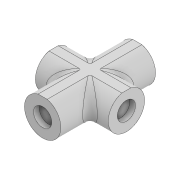
# Autodesk Inventor part: Cross_Minimo
Saved by Autodesk Inventor 2020 (Build 240168000, 168)
## iProperties
Created: 2021-03-31
Part Number: Cross_Minimo
Material: Generic
Document SubType Name: Modeling
Designer: deox
Density: 1 g/cm^3
Appearance: Default
Author: deox
## iProperties of the stored document _3DPrint.ipt
Created: 2021-05-12
Part Number: _3DPrint
Material: Generic
Document SubType Name: Modeling
Designer: deox
Density: 1 g/cm^3
Appearance: Default
Author: deox
Autodesk Inventor part; units mm, degrees
ref_plane "YZ Plane" through (0, 0, 0) normal (1, 0, 0) x (0, 1, 0)
ref_plane "XZ Plane" through (0, 0, 0) normal (0, 1, 0) x (-1, 0, 0)
ref_plane "XY Plane" through (0, 0, 0) normal (0, 0, 1) x (1, 0, 0)
sketch "Sketch1" plane through (0, 0, 0) normal (0, 0, 1) x (1, 0, 0)
  circle A0 centre (0, 0) radius 2.5
  dimension "d0" = 5
  constraints: 1 centre point, 1 coincident
  measures "d0" diameter of A0
extrude "Extrusion1" add sketch "Sketch1" along normal mid plane 13
sketch "Sketch2" plane through (0, 0, 6.5) normal (0, 0, 1) x (1, 0, 0)
  circle A0 centre (0, 0) radius 1.25
  dimension "d3" = 2.5
  constraints: 1 centre point, 1 coincident
  measures "d3" diameter of A0
extrude "Extrusion2" cut sketch "Sketch2" against normal blind 0.8
mirror "Mirror1" about plane through (0, 0, 0) normal (0, 0, 1) of "Extrusion2"
sketch "Sketch3" plane through (0, 0, 0) normal (1, 0, 0) x (0, 1, 0)
  circle A0 centre (0, 0) radius 2.5
  dimension "d6" = 5
  constraints: 1 centre point, 1 coincident
  measures "d6" diameter of A0
extrude "Extrusion3" add sketch "Sketch3" along normal mid plane 10
sketch "Sketch4" plane through (5, 0, 0) normal (1, 0, 0) x (0, 0, -1)
  circle A0 centre (0, 0) radius 1.25
  dimension "d9" = 2.5
  constraints: 1 centre point, 1 coincident
  measures "d9" diameter of A0
extrude "Extrusion4" cut sketch "Sketch4" against normal blind 0.8
mirror "Mirror2" about plane through (0, 0, 0) normal (1, 0, 0) of "Extrusion4"
fillet "Fillet1" radius 1 6 edges at (1.7678, 1.7678, 1.7678) (-2.5, 0, 2.5) (1.7678, -1.7678, 1.7678) (1.7678, -1.7678, -1.7678) (1.7678, 1.7678, -1.7678) (-2.5, 0, -2.5)
sketch "Sketch5" plane through (0, 0, 6.5) normal (0, 0, 1) x (1, 0, 0)
  circle A0 centre (0, 0) radius 2.5 projected
  line L0 (0, 2.5) -> (5.3723, 2.5)
  line L1 (5.3723, 2.5) -> (5.3723, 2.4205)
  line L2 (5.3723, 2.4205) -> (0, 2.4205)
  line L3 (0, 2.4205) -> (0, 2.5)
  line L4 (0, 2.5) -> (-5.4474, 2.5)
  line L5 (-5.4474, 2.5) -> (-5.4474, 2.4205)
  line L6 (-5.4474, 2.4205) -> (0, 2.4205)
  line L7 (0, 2.4205) -> (0, 2.5)
  constraints: 16 end point, 4 parallel, 2 horizontal, 2 perpendicular, 1 point on line, 1 vertical alignment, 1 other
extrude "Extrusion5" cut sketch "Sketch5" against normal through all contours L2 L3 A0 | A0 L0 L1 L2 | L6 L5 L4 A0 | A0 L3 L6
ref_plane "Work Plane1" through (0, 0, 0) normal (0, 0, 1) x (1, 0, 0)
body "Solid1"
